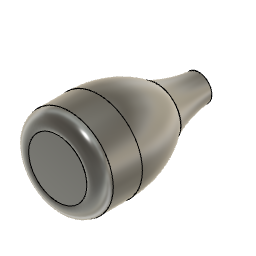
Semana2_desafio4 (Autodesk Fusion 360 design; units mm, degrees)
Autodesk Fusion 360 part; units mm, degrees
sketch "Sketch1" plane through (0, 0, 0) normal (0, 0, 1) x (1, 0, 0)
  line L0 (50, 13) -> (60, 13) construction
  arc A0 (33, 0) -> (50, 13) centre (36.5294, 13) ccw
  line L1 (0, 0) -> (33, 0)
  line L2 (50, 13) -> (50, 50) construction
  arc A1 (15, 160) -> (27.5263, 112.4106) centre (160.6332, 172.8898) ccw
  line L3 (50, 46.1163) -> (50, 13)
  arc A2 (50, 46.1163) -> (27.5263, 112.4106) centre (-59.0164, 46.1163) ccw
  line L4 (0, 0) -> (0, 159)
  spline S0 degree 5 poles (15, 160) (14.8262, 159.9413) (14.4709, 159.828) (13.9149, 159.6701) (13.1268, 159.4837) (12.0634, 159.2918) (10.9233, 159.1418) (9.7131, 159.0335) (8.4465, 158.9651) (7.1479, 158.9321) (5.8529, 158.927) (4.6023, 158.9413) (3.4386, 158.9657) (2.4011, 158.9914) (1.5217, 159.0114) (0.8187, 159.021) (0.4012, 159.0189) (0.1693, 159.0117) (0.0505, 159.0043) (0, 159) knots 0 0 0 0 0 0 0.066667 0.133333 0.2 0.266667 0.333333 0.4 0.466667 0.533333 0.6 0.666667 0.733333 0.8 0.866667 0.933333 1 1 1 1 1 1
  arc A3 (14.228, 158.8592) -> (26.7725, 111.9582) centre (160.6332, 172.8898) ccw
  arc A4 (49.1266, 46.1163) -> (26.7725, 111.9582) centre (-59.0164, 46.1163) ccw
  line L5 (49.1266, 46.1163) -> (49.1266, 13)
  arc A5 (33.1184, 0.8734) -> (49.1266, 13) centre (36.5294, 13) ccw
  line L6 (0.8734, 0.8734) -> (33.1184, 0.8734)
  line L7 (14.228, 158.8592) -> (14.1436, 159.7405)
  line L8 (0.8734, 0.8734) -> (0, 0.8734)
  point P0 (9, 159)
  point P1 (2, 159)
  dimension "d4" = 13
  dimension "d5" = 13.4706
  dimension "d6" = 70
  constraint coincident L1.start L4.start
  constraint horizontal L1
  constraint perpendicular L0 L2
  constraint perpendicular L1 L4
  constraint coincident S0 L7.end
  constraint tangent A3 L7
  constraint concentric A1 A3
  constraint concentric A2 A4
  constraint parallel L3 L5
  constraint concentric A0 A5
  constraint parallel L1 L6
  constraint tangent A4 L5
  constraint tangent L5 A5
  constraint coincident L4 L8.end
  constraint perpendicular L4 L8
  measures "d4" distance of L0 L1
  measures "d5" radius of A0
  measures "d6" distance of L3.start A1.end
revolve "Revolve1" add sketch "Sketch1" angle 360 about axis through (0, 0, 0) along (0, 1, 0) contours A0 L1 A1 L3 A2 L4 S0 A3 A4 L5 A5 L6 L7 L8
